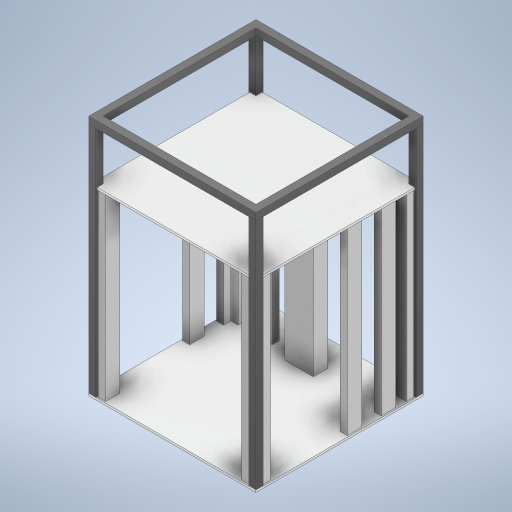
# Autodesk Inventor part: RevIII Refined Printer Envelope Study
Saved by Autodesk Inventor 2024 (Build 280153000, 153)
## iProperties
Created: 2024-07-28
Part Number: RevIII Refined Printer Envelope Study
Material: Generic
Document SubType Name: Modeling
Designer: Ishaan
Density: 1 g/cm^3
Appearance: Default
Author: Ishaan
Autodesk Inventor part; units mm, degrees
ref_plane "YZ Plane" through (0, 0, 0) normal (1, 0, 0) x (0, 1, 0)
ref_plane "XZ Plane" through (0, 0, 0) normal (0, 1, 0) x (-1, 0, 0)
ref_plane "XY Plane" through (0, 0, 0) normal (0, 0, 1) x (1, 0, 0)
sketch "Sketch1" plane through (0, 0, 0) normal (0, 0, 1) x (1, 0, 0)
  line L0 (233.25, -233.25) -> (-233.25, -233.25)
  line L1 (-233.25, -233.25) -> (-233.25, 233.25)
  line L2 (-233.25, 233.25) -> (233.25, 233.25)
  line L3 (233.25, 233.25) -> (233.25, -233.25)
  line L4 (233.25, -233.25) -> (-233.25, 233.25) construction
  line L5 (-233.25, -233.25) -> (233.25, 233.25) construction
  line L6 (-233.25, 233.25) -> (-213.25, 233.25)
  line L7 (-213.25, 233.25) -> (-213.25, 213.25)
  line L8 (-213.25, 213.25) -> (-233.25, 213.25)
  line L9 (-233.25, 213.25) -> (-233.25, 233.25)
  line L10 (233.25, 233.25) -> (213.25, 233.25)
  line L11 (213.25, 233.25) -> (213.25, 213.25)
  line L12 (213.25, 213.25) -> (233.25, 213.25)
  line L13 (233.25, 213.25) -> (233.25, 233.25)
  line L14 (-233.25, -233.25) -> (-213.25, -233.25)
  line L15 (-213.25, -233.25) -> (-213.25, -213.25)
  line L16 (-213.25, -213.25) -> (-233.25, -213.25)
  line L17 (-233.25, -213.25) -> (-233.25, -233.25)
  line L18 (233.25, -233.25) -> (213.25, -233.25)
  line L19 (213.25, -233.25) -> (213.25, -213.25)
  line L20 (213.25, -213.25) -> (233.25, -213.25)
  line L21 (233.25, -213.25) -> (233.25, -233.25)
  line L22 (-190, 190) -> (-210, 190)
  line L23 (-210, 190) -> (-210, 230)
  line L24 (-210, 230) -> (-190, 230)
  line L25 (-190, 230) -> (-190, 190)
  line L26 (-190, 190) -> (-230, 190)
  line L27 (-230, 190) -> (-230, 210)
  line L28 (-230, 210) -> (-190, 210)
  line L29 (-190, 210) -> (-190, 190)
  line L30 (190, 230) -> (210, 230)
  line L31 (210, 230) -> (210, 190)
  line L32 (210, 190) -> (190, 190)
  line L33 (190, 190) -> (190, 230)
  line L34 (190, 190) -> (230, 190)
  line L35 (230, 190) -> (230, 210)
  line L36 (230, 210) -> (190, 210)
  line L37 (190, 210) -> (190, 190)
  line L38 (-230, -190) -> (-190, -190)
  line L39 (-190, -190) -> (-190, -210)
  line L40 (-190, -210) -> (-230, -210)
  line L41 (-230, -210) -> (-230, -190)
  line L42 (-190, -190) -> (-210, -190)
  line L43 (-210, -190) -> (-210, -230)
  line L44 (-210, -230) -> (-190, -230)
  line L45 (-190, -230) -> (-190, -190)
  line L46 (190, -190) -> (230, -190)
  line L47 (230, -190) -> (230, -210)
  line L48 (230, -210) -> (190, -210)
  line L49 (190, -210) -> (190, -190)
  line L50 (190, -190) -> (210, -190)
  line L51 (210, -190) -> (210, -230)
  line L52 (210, -230) -> (190, -230)
  line L53 (190, -230) -> (190, -190)
  line L54 (-40, 160) -> (40, 160)
  line L55 (40, 160) -> (40, 120)
  line L56 (40, 120) -> (-40, 120)
  line L57 (-40, 120) -> (-40, 160)
  circle A0 centre (-112.5, -82.5) radius 105
  circle A1 centre (112.5, -82.5) radius 105
  line L58 (-112.5, -82.5) -> (112.5, -82.5) construction
  line L59 (150, -180) -> (-150, -180)
  line L60 (-150, -180) -> (-150, 70)
  line L61 (-150, 70) -> (150, 70)
  line L62 (150, 70) -> (150, -180)
  line L63 (150, -180) -> (-150, 70) construction
  line L64 (-150, -180) -> (150, 70) construction
  line L65 (-230, 160) -> (-210, 160)
  line L66 (-210, 160) -> (-210, 120)
  line L67 (-210, 120) -> (-230, 120)
  line L68 (-230, 120) -> (-230, 160)
  line L69 (-230, 160) -> (-190, 160)
  line L70 (-190, 160) -> (-190, 140)
  line L71 (-190, 140) -> (-230, 140)
  line L72 (-230, 140) -> (-230, 160)
  line L73 (-135, 160) -> (-95, 160)
  line L74 (-95, 160) -> (-95, 140)
  line L75 (-95, 140) -> (-135, 140)
  line L76 (-135, 140) -> (-135, 160)
  line L77 (-230, 65) -> (-210, 65)
  line L78 (-210, 65) -> (-210, 25)
  line L79 (-210, 25) -> (-230, 25)
  line L80 (-230, 25) -> (-230, 65)
  line L81 (-210, 25) -> (-210, -190) construction
  line L82 (95, 160) -> (135, 160)
  line L83 (135, 160) -> (135, 140)
  line L84 (135, 140) -> (95, 140)
  line L85 (95, 140) -> (95, 160)
  line L86 (230, 140) -> (190, 140)
  line L87 (190, 140) -> (190, 160)
  line L88 (190, 160) -> (230, 160)
  line L89 (230, 160) -> (230, 140)
  line L90 (230, 160) -> (210, 160)
  line L91 (210, 160) -> (210, 120)
  line L92 (210, 120) -> (230, 120)
  line L93 (230, 120) -> (230, 160)
  line L94 (230, 65) -> (210, 65)
  line L95 (210, 65) -> (210, 25)
  line L96 (210, 25) -> (230, 25)
  line L97 (230, 25) -> (230, 65)
  point P0 (0, 0)
  point P1 (0, 233.25)
  point P2 (0, 160)
  point P3 (0, -82.5)
  point P4 (0, -55)
  point P5 (0, 70)
  point P6 (-210, -82.5)
  point P7 (-210, 140)
  point P8 (-210, 210)
  point P9 (210, 210)
  point P10 (210, 140)
  point P11 (210, -210)
  point P12 (-210, -210)
  dimension "d0" = 466.5
  dimension "d1" = 466.5
  dimension "d2" = 20
  dimension "d3" = 20
  dimension "d6" = 20
  dimension "d7" = 40
  dimension "d8" = 3.25
  dimension "d9" = 3.25
  dimension "d10" = 3.25
  dimension "d11" = 3.25
  dimension "d12" = 3.25
  dimension "d13" = 3.25
  dimension "d14" = 3.25
  dimension "d15" = 3.25
  dimension "d16" = 80
  dimension "d17" = 40
  dimension "d19" = 70
  dimension "d20" = 210
  dimension "d21" = 210
  dimension "d22" = 225
  dimension "d26" = 300
  dimension "d27" = 250
  dimension "d28" = 50
  dimension "d29" = 150
  dimension "d30" = 40
  dimension "d31" = 20
  dimension "d32" = 55
  dimension "d33" = 55
  dimension "d36" = 55
  dimension "d37" = 55
  constraints: 196 end point, 46 parallel, 34 equal length, 24 horizontal, 23 perpendicular, 9 collinear, 9 midpoint, 3 vertical alignment, 2 centre point, 1 point on line
  measures "d0" distance of L1.end L2.end
  measures "d1" distance of L0.end L1.end
  measures "d2" distance of L7.end L8.end
  measures "d3" distance of L6.end L7.end
  measures "d6" distance of L23.end L24.end
  measures "d7" distance of L24.end L22.start
  measures "d8" distance between parallel lines of L23 L7
  measures "d9" distance between parallel lines of L28 L8
  measures "d10" distance between parallel lines of L12 L36
  measures "d11" distance between parallel lines of L11 L31
  measures "d12" distance between parallel lines of L40 L16
  measures "d13" distance between parallel lines of L15 L43
  measures "d14" distance between parallel lines of L19 L51
  measures "d15" distance between parallel lines of L48 L20
  measures "d16" distance of L55.end L56.end
  measures "d17" distance of L54.end L55.end
  measures "d19" distance between parallel lines of L30 L54
  measures "d20" diameter of A0
  measures "d21" diameter of A1
  measures "d22" distance of L58.start L58.end
  measures "d26" distance of L60.end L61.end
  measures "d27" distance of L59.end L60.end
  measures "d28" distance between parallel lines of L61 L56
  measures "d29" distance between parallel lines of L57 L70
  measures "d30" distance of L74.end L75.end
  measures "d31" distance of L73.end L74.end
  measures "d32" distance between parallel lines of L76 L70
  measures "d33" distance between parallel lines of L57 L74
  measures "d36" distance between parallel lines of L77 L67
  measures "d37" distance between parallel lines of L85 L55
extrude "Extrusion1" add sketch "Sketch1" against normal blind 6.35 contours L0 L19 L20 L3 | L0 L15 L16 L1 L8 L7 L2 L11 L12 L3 L20 L19 | L0 L1 L16 L15 | L12 L11 L2 L3 | L1 L2 L7 L8 | L22 L23 L28 L25 | L26 L27 L28 L23 | L28 L23 L24 L25 | L30 L31 L36 L33 | L36 L31 L32 L33 | L36 L35 L34 L31 | L38 L43 L40 L41 | L38 L39 L40 L43 | L40 L45 L44 L43 | L46 L51 L48 L49 | L46 L47 L48 L51 | L48 L51 L52 L53 | L54 L55 L56 L57 | A0 L59 L60 | A0 L60 L61 L62 A1 L59 | L60 L59 A0 | L59 L62 A1 | A1 L62 L59 | L65 L66 L71 L68 | L69 L70 L71 L66 | L71 L66 L67 L68 | L73 L74 L75 L76 | L77 L78 L79 L80 | L82 L83 L84 L85 | L93 L92 L91 L86 | L86 L91 L88 L89 | L86 L87 L88 L91 | L97 L96 L95 L94
extrude "Extrusion2" add sketch "Sketch1" along normal blind 500 separate body contours L22 L23 L28 L25 | L26 L27 L28 L23 | L28 L23 L24 L25 | L30 L31 L36 L33 | L36 L31 L32 L33 | L36 L35 L34 L31 | L38 L43 L40 L41 | L38 L39 L40 L43 | L40 L45 L44 L43 | L46 L51 L48 L49 | L46 L47 L48 L51 | L48 L51 L52 L53 | L54 L55 L56 L57 | L65 L66 L71 L68 | L69 L70 L71 L66 | L71 L66 L67 L68 | L73 L74 L75 L76 | L77 L78 L79 L80 | L82 L83 L84 L85 | L93 L92 L91 L86 | L86 L91 L88 L89 | L86 L87 L88 L91 | L97 L96 L95 L94
sketch "Sketch2" plane through (0, 0, 500) normal (0, 0, 1) x (1, 0, 0)
  line L0 (230, 210) -> (210, 210) projected
  line L1 (210, 210) -> (210, 230) projected
  line L2 (210, 230) -> (190, 230) projected
  line L3 (190, 230) -> (190, 190) projected
  line L4 (190, 190) -> (230, 190) projected
  line L5 (230, 190) -> (230, 210) projected
  line L6 (210, -230) -> (210, -210) projected
  line L7 (210, -210) -> (230, -210) projected
  line L8 (230, -210) -> (230, -190) projected
  line L9 (230, -190) -> (190, -190) projected
  line L10 (190, -190) -> (190, -230) projected
  line L11 (190, -230) -> (210, -230) projected
  line L12 (-230, -210) -> (-210, -210) projected
  line L13 (-210, -210) -> (-210, -230) projected
  line L14 (-210, -230) -> (-190, -230) projected
  line L15 (-190, -230) -> (-190, -190) projected
  line L16 (-190, -190) -> (-230, -190) projected
  line L17 (-230, -190) -> (-230, -210) projected
  line L18 (-210, 230) -> (-210, 210) projected
  line L19 (-210, 210) -> (-230, 210) projected
  line L20 (-230, 210) -> (-230, 190) projected
  line L21 (-230, 190) -> (-190, 190) projected
  line L22 (-190, 190) -> (-190, 230) projected
  line L23 (-190, 230) -> (-210, 230) projected
  line L24 (230, 230) -> (-230, 230)
  line L25 (-230, 230) -> (-230, -230)
  line L26 (-230, -230) -> (230, -230)
  line L27 (230, -230) -> (230, 230)
  line L28 (190, -230) -> (210, -230) projected
  line L29 (230, -210) -> (230, -190) projected
  line L30 (210, 230) -> (190, 230) projected
  line L31 (-230, 210) -> (-230, 190) projected
  line L32 (-233.25, 233.25) -> (233.25, 233.25) projected
  line L33 (-233.25, 233.25) -> (-213, 233.25)
  line L34 (-213, 233.25) -> (-213, 213)
  line L35 (-213, 213) -> (-233.25, 213)
  line L36 (-233.25, 213) -> (-233.25, 233.25)
  line L37 (233.25, 233.25) -> (213, 233.25)
  line L38 (213, 233.25) -> (213, 213)
  line L39 (213, 213) -> (233.25, 213)
  line L40 (233.25, 213) -> (233.25, 233.25)
  line L41 (233.25, -233.25) -> (213, -233.25)
  line L42 (213, -233.25) -> (213, -213)
  line L43 (213, -213) -> (233.25, -213)
  line L44 (233.25, -213) -> (233.25, -233.25)
  line L45 (-233.25, -233.25) -> (-213, -233.25)
  line L46 (-213, -233.25) -> (-213, -213)
  line L47 (-213, -213) -> (-233.25, -213)
  line L48 (-233.25, -213) -> (-233.25, -233.25)
  line L49 (-233.25, -233.25) -> (233.25, -233.25) projected
  point P0 (-230, -213)
  point P1 (-213, -230)
  point P2 (230, -213)
  point P3 (213, -230)
  point P4 (230, 213)
  point P5 (213, 230)
  point P6 (-230, 213)
  point P7 (-213, 230)
  dimension "d44" = 20.25
  dimension "d45" = 20.25
  constraints: 40 end point, 10 parallel, 6 equal length, 5 collinear, 5 horizontal, 5 perpendicular, 3 point on line
  measures "d44" distance of L34.end L35.end
  measures "d45" distance of L33.end L34.end
extrude "Extrusion3" add sketch "Sketch2" along normal blind 6.35 separate body contours L5 L4 L3 L2 L1 L0 | L0 L1 L24 L38 L39 L27 | L27 L9 L10 L26 L15 L16 L25 L21 L22 L24 L3 L4 | L8 L7 L6 L11 L10 L9 | L27 L43 L42 L26 L6 L7 | L22 L21 L20 L19 L18 L23 | L18 L19 L25 L35 L34 L24 | L14 L13 L12 L17 L16 L15 | L26 L46 L47 L25 L12 L13
extrude "Extrusion4" add sketch "Sketch1" along normal blind 650 separate body contours L0 L19 L20 L3 | L0 L1 L16 L15 | L12 L11 L2 L3 | L1 L2 L7 L8
sketch "Sketch3" plane through (0, 0, 650) normal (0, 0, 1) x (1, 0, 0)
  line L0 (-233.25, -213.25) -> (-233.25, -233.25) projected
  line L1 (-233.25, -233.25) -> (-213.25, -233.25) projected
  line L2 (-213.25, -233.25) -> (-213.25, -213.25) projected
  line L3 (-213.25, -213.25) -> (-233.25, -213.25) projected
  line L4 (-213.25, 213.25) -> (-213.25, 233.25) projected
  line L5 (-213.25, 233.25) -> (-233.25, 233.25) projected
  line L6 (-233.25, 233.25) -> (-233.25, 213.25) projected
  line L7 (-233.25, 213.25) -> (-213.25, 213.25) projected
  line L8 (233.25, 213.25) -> (233.25, 233.25) projected
  line L9 (233.25, 233.25) -> (213.25, 233.25) projected
  line L10 (213.25, 233.25) -> (213.25, 213.25) projected
  line L11 (213.25, 213.25) -> (233.25, 213.25) projected
  line L12 (213.25, -213.25) -> (213.25, -233.25) projected
  line L13 (213.25, -233.25) -> (233.25, -233.25) projected
  line L14 (233.25, -233.25) -> (233.25, -213.25) projected
  line L15 (233.25, -213.25) -> (213.25, -213.25) projected
  line L16 (233.25, -233.25) -> (-233.25, -233.25)
  line L17 (-233.25, -233.25) -> (-233.25, 233.25)
  line L18 (-233.25, 233.25) -> (233.25, 233.25)
  line L19 (233.25, 233.25) -> (233.25, -233.25)
  line L20 (-213.25, 213.25) -> (213.25, 213.25)
  line L21 (213.25, 213.25) -> (213.25, -213.25)
  line L22 (213.25, -213.25) -> (-213.25, -213.25)
  line L23 (-213.25, -213.25) -> (-213.25, 213.25)
  point P0 (0, 0)
  constraints: 16 end point, 4 parallel, 2 horizontal, 2 perpendicular
extrude "Extrusion5" add sketch "Sketch3" along normal blind 20 separate body contours L3 L2 L1 L0 | L17 L7 L23 L3 | L22 L12 L16 L2 | L6 L5 L4 L7 | L15 L14 L13 L12 | L21 L11 L19 L15 | L4 L18 L10 L20 | L10 L9 L8 L11
equation "\"d1\" = d0"
equation "\"d10\" = d9"
equation "\"d11\" = d10"
equation "\"d12\" = d9"
equation "\"d13\" = d8"
equation "\"d14\" = d13"
equation "\"d15\" = d12"
equation "\"d32\" = d33"
equation "\"d36\" = d32"
equation "\"d37\" = d33"
body "Solid1"
body "Solid2"
body "Solid3"
body "Solid4"
body "Solid5"
